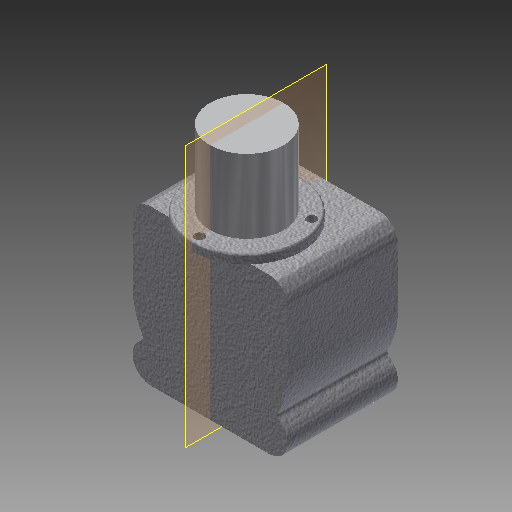
# Autodesk Inventor part: Pneumatics_VIAIR_0090_02
Saved by Autodesk Inventor 2017 (Build 210142000, 142)
## iProperties
Created: 2011-02-24
Part Number: Pneumatics_VIAIR_0090_02
Document SubType Name: Modeling
Designer: s-2512184
Density: 1 g/cm^3
Description: AIR COMPRESSOR END 2
Vendor: VIAIR
Material: Generic
Appearance: Aluminum Cast
Author: s-2512184
Title: AIR COMPRESSOR END 2
Autodesk Inventor part; units mm, degrees
note: some values were not read from the file. Chosen so that the rebuilt part matches the saved one: sketch regions of "Extrusion2".
ref_plane "XZ Plane" through (0, 0, 0) normal (0, 1, 0) x (-1, 0, 0)
ref_plane "XY Plane" through (0, 0, 0) normal (0, 0, 1) x (1, 0, 0)
sketch "Sketch1" plane through (0, 0, 0) normal (0, 0, 1) x (1, 0, 0)
  line L0 (-26.797, 26.797) -> (26.797, 26.797)
  line L1 (26.797, 26.797) -> (26.797, -26.797)
  line L2 (26.797, -26.797) -> (-26.797, -26.797)
  line L3 (-26.797, -26.797) -> (-26.797, 26.797)
  point P0 (0, 0)
  point P1 (-26.797, 0)
  point P2 (0, 26.797)
  dimension "d0" = 53.594
  dimension "d1" = 53.594
  constraints: 8 end point, 2 midpoint, 2 parallel, 1 horizontal, 1 horizontal alignment, 1 perpendicular, 1 vertical alignment
  measures "d0" distance of L1.end L2.end
  measures "d1" distance of L0.end L1.end
extrude "Extrusion1" add sketch "Sketch1" along normal blind 38.1
fillet "Fillet1" radius 6.35 2 edges at (-26.797, 26.797, 19.05) (26.797, 26.797, 19.05)
sketch "Sketch3" plane through (0, 0, 38.1) normal (0, 0, 1) x (1, 0, 0)
  arc A0 (26.797, 20.447) -> (20.447, 26.797) centre (20.447, 20.447) ccw projected
  line L0 (-20.447, 26.797) -> (20.447, 26.797) projected
  arc A1 (-20.447, 26.797) -> (-26.797, 20.447) centre (-20.447, 20.447) ccw projected
  line L1 (-26.797, -26.797) -> (-26.797, 20.447) projected
  line L2 (26.797, -26.797) -> (-26.797, -26.797) projected
  line L3 (26.797, 20.447) -> (26.797, -26.797) projected
  arc A2 (-22.5612, -14.4593) -> (-20.447, -26.797) centre (-20.447, -20.447) ccw
  arc A3 (20.447, -26.797) -> (22.5612, -14.4593) centre (20.447, -20.447) ccw
  line L4 (-26.797, -26.797) -> (26.797, -26.797)
  line L5 (-26.797, 0) -> (-26.797, -26.797)
  line L6 (26.797, 0) -> (26.797, -26.797)
  arc A4 (22.5612, -14.4593) -> (-22.5612, -14.4593) centre (0, 0) ccw
  line L7 (-26.797, 0) -> (-26.797, 20.447)
  line L8 (-20.447, 26.797) -> (20.447, 26.797)
  line L9 (26.797, 20.447) -> (26.797, 0)
  arc A5 (-20.447, 26.797) -> (-26.797, 20.447) centre (-20.447, 20.447) ccw
  arc A6 (26.797, 20.447) -> (20.447, 26.797) centre (20.447, 20.447) ccw
  dimension "d9" = 12.7
  dimension "d10" = 12.7
  dimension "d12" = 26.797
  constraints: 12 end point, 12 point on circle, 8 tangent, 5 centre point, 4 collinear, 4 point on line, 1 coincident, 1 concentric
  measures "d9" diameter of A2
  measures "d10" diameter of A3
  measures "d12" radius of A4
extrude "Extrusion2" cut sketch "Sketch3" against normal through all contours L3 A3 A4 | L3 L2 A3 | A4 A2 L1 | A2 L2 L1
fillet "Fillet2" radius 1.5875 2 edges at (22.5612, -14.4593, 19.05) (-22.5612, -14.4593, 19.05)
sketch "Sketch4" plane through (-20.447, 26.797, 0) normal (0, 1, 0) x (1, 0, 0)
  line L0 (0, 0) -> (40.894, 0) projected
  line L1 (-6.35, -38.1) -> (0, -38.1) projected
  line L2 (0, -38.1) -> (0, 0) projected
  line L3 (0, 0) -> (-6.35, 0) projected
  line L4 (-6.35, 0) -> (-6.35, -38.1) projected
  line L5 (43.8591, 0) -> (43.8591, -38.1) projected
  line L6 (40.894, -38.1) -> (47.244, -38.1) projected
  line L7 (47.244, -38.1) -> (47.244, 0) projected
  line L8 (47.244, 0) -> (40.894, 0) projected
  line L9 (40.894, 0) -> (40.894, -38.1) projected
  line L10 (-2.9651, -38.1) -> (-2.9651, 0) projected
  circle A0 centre (20.447, -25.4) radius 19.05
  point P0 (20.447, 0)
  point P1 (20.447, -6.35)
  point P2 (20.447, 0)
  dimension "d16" = 38.1
  dimension "d17" = 6.35
  constraints: 3 vertical alignment, 1 midpoint, 2 other
  measures "d17" distance from line of L0 point (20.447, -6.35)
extrude "Extrusion3" add sketch "Sketch4" along normal blind 3.175 contours A0
fillet "Fillet3" radius 0.7937 1 edges at (-19.05, 29.972, 25.4)
sketch "Sketch5" plane through (0, 29.972, 25.4) normal (0, 1, 0) x (1, 0, 0)
  circle A0 centre (0, 0) radius 18.2562 projected
  circle A1 centre (0, 0) radius 12.7
  circle A2 centre (0, 0) radius 19.05 projected
  point P0 (0, 25.4)
  dimension "d24" = 6.35
  constraints: 1 centre point, 1 coincident
  measures "d24" radial gap between concentric circles of A2 A1
extrude "Extrusion4" add sketch "Sketch5" along normal blind 25.4 contours A1
sketch "Sketch6" plane through (0, 29.972, 25.4) normal (0, 1, 0) x (1, 0, 0)
  circle A0 centre (-14.1881, 8.1915) radius 1.6383 projected
  circle A1 centre (0, -16.383) radius 1.6383 projected
  circle A2 centre (14.1881, 8.1915) radius 1.6383 projected
  point P0 (0, 25.4)
hole "Hole1" at (0, 29.972, 41.783) at (14.1881, 29.972, 17.2085) at (-14.1881, 29.972, 17.2085) direction (0, -1, 0) diameter 3.2766 depth 6.35 tip angle 118 clearance for "Flat Head Machine Screw (82)" size "#4" standard "Ansi Unified Screw Threads"
body "Solid1"
